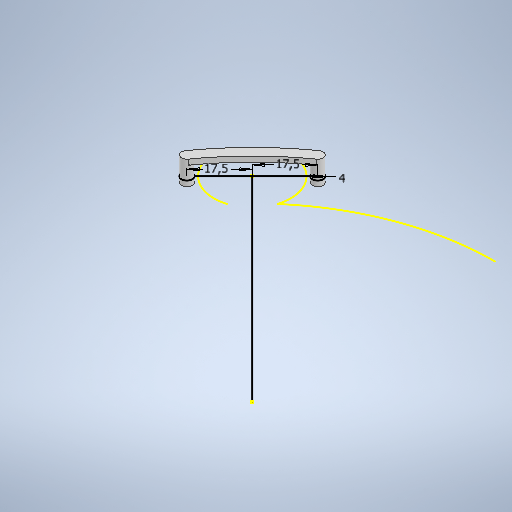
# Autodesk Inventor part: uchwyt
Saved by Autodesk Inventor 2025 (Build 290162000, 162)
## iProperties
Created: 2025-01-24
Part Number: uchwyt
Material: Generic
Document SubType Name: Modeling
Designer: piotr
Density: 1 g/cm^3
Appearance: Default
Author: piotr
Autodesk Inventor part; units mm, degrees
ref_plane "YZ Plane" through (0, 0, 0) normal (1, 0, 0) x (0, 1, 0)
ref_plane "XZ Plane" through (0, 0, 0) normal (0, 1, 0) x (-1, 0, 0)
ref_plane "XY Plane" through (0, 0, 0) normal (0, 0, 1) x (1, 0, 0)
sketch "Sketch3" plane through (0, 0, 0) normal (0, 1, 0) x (-1, 0, 0)
  circle A0 centre (0, 0) radius 91.797
  circle A1 centre (0, 0) radius 110.99
  line L0 (0, 0) -> (110.99, 0)
  line L1 (0, 0) -> (0, -110.99)
  line L2 (91.797, 0) -> (110.99, 0)
  line L3 (0, -45.742) -> (0, -110.99)
  circle A2 centre (0, -101.3935) radius 9.5965
  circle A3 centre (101.3935, 0) radius 9.5965
  circle A4 centre (101.3935, 0) radius 3.125
  circle A5 centre (0, -101.3935) radius 3.125
  circle A6 centre (0, 0) radius 130.99
  line L4 (0, 0) -> (119.0731, -119.0731)
  line L5 (64.9103, -64.9103) -> (73.8174, -73.8174)
  circle A7 centre (73.8174, -73.8174) radius 14.5
  line L6 (76.1136, -88.1344) -> (88.1344, -76.1136)
  line L7 (76.1136, -88.1344) -> (80.7098, -92.7306)
  line L8 (88.1344, -76.1136) -> (92.7306, -80.7098)
  line L9 (80.7098, -92.7306) -> (92.7306, -80.7098)
  line L10 (73.8174, -73.8174) -> (80.7098, -66.9249)
  line L11 (57.15, -95.1455) -> (82.124, -102.0492)
  line L12 (95.1455, -57.15) -> (102.0492, -82.124)
  point P0 (0, -91.797)
  point P1 (103.6367, -80.1113)
  point P2 (69.4945, -59.9767)
  point P3 (87.3148, -68.5194)
  point P4 (68.5194, -87.3148)
  point P5 (59.9767, -69.4945)
  dimension "d9" = 183.594
  dimension "d10" = 221.98
  dimension "d11" = 6.25
  dimension "d14" = 6.25
  dimension "d20" = 20
  dimension "d29" = 45
  dimension "d30" = 12.5965
  dimension "d31" = 29
  dimension "d32" = 17
  dimension "d33" = 6.5
  dimension "d34" = 6.5
  constraints: 26 end point, 9 point on circle, 8 centre point, 5 coincident, 5 perpendicular, 5 point on line, 4 tangent, 2 collinear, 2 symmetric about line, 1 horizontal, 1 midpoint
  measures "d9" diameter of A0
  measures "d10" diameter of A1
  measures "d11" diameter of A4
  measures "d14" diameter of A5
  measures "d20" radial gap between concentric circles of A1 A6
  measures "d29" angle of L4 L1
  measures "d30" distance of L5.start L5.end
  measures "d31" diameter of A7
  measures "d32" distance of L6.start L6.end
  measures "d33" distance of L6.start L7.end
  measures "d34" distance of L6.end L8.end
extrude "Extrusion2" add sketch "Sketch3" along normal blind 3 contours A3 A1 A7 A0 | A3 L0 A4 | L0 A4 A3 | A2 L1 A5 | A0 A7 A1 A2 | L1 A5 A2
extrude "Extrusion3" add sketch "Sketch3" along normal blind 2 contours A1 L12 A6 L4 L9 L8 A7 | A7 L7 L9 L4 A6 L11 A1
fillet "Fillet8" radius 0.99 7 edges at (-62.9566, 2, -91.4071) (-57.15, 1, -95.1455) (-91.4071, 2, -62.9566) (-95.1455, 1, -57.15) (-69.637, 2, -98.5973) (-92.6239, 2, -92.6239) (-98.5973, 2, -69.637)
chamfer "Chamfer2" distance 2 angle 45 1 edges at (-86.7202, 2, -86.7202)
sketch "Sketch5" plane through (0, 3, 0) normal (0, 1, 0) x (1, 0, 0)
  arc A0 (-59.9767, 69.4945) -> (-68.5194, 87.3148) centre (-73.8174, 73.8174) ccw projected
  arc A1 (-87.3148, 68.5194) -> (-69.4945, 59.9767) centre (-73.8174, 73.8174) ccw projected
  arc A2 (0, 91.797) -> (-59.9767, 69.4945) centre (0, 0) ccw projected
  line L0 (0, 0) -> (-73.8174, 73.8174)
  line L1 (-61.443, 86.1917) -> (-73.8174, 73.8174)
  line L2 (-73.8174, 73.8174) -> (-86.1917, 61.443)
  circle A3 centre (-61.443, 86.1917) radius 2
  circle A4 centre (-86.1917, 61.443) radius 2
  dimension "d45" = 17.5
  dimension "d46" = 17.5
  dimension "d47" = 4
  constraints: 6 end point, 2 centre point, 2 coincident, 1 perpendicular, 1 point on line, 1 symmetric about line, 1 other
  measures "d45" distance of L1.start L1.end
  measures "d46" distance of L1.end L2.end
  measures "d47" diameter of A3
extrude "Extrusion4" cut sketch "Sketch5" against normal blind 10
extrude "Extrusion5" add sketch "Sketch5" along normal blind 5 separate body
sketch "Sketch6" plane through (-86.1917, 8, -61.443) normal (0, 1, 0) x (1, 0, 0)
  circle A0 centre (86.1917, -61.443) radius 107.8501
  circle A1 centre (24.7487, 24.7487) radius 2 projected
  circle A2 centre (86.1917, -61.443) radius 103.8501
  circle A3 centre (0, 0) radius 2 projected
  point P0 (1.6286, -1.1609)
  point P1 (25.9097, 23.1202)
  point P2 (23.5878, 26.3773)
  point P3 (-1.6286, 1.1609)
  constraints: 3 tangent, 2 centre point, 2 coincident
extrude "Extrusion6" add sketch "Sketch6" along normal blind 2 contours A1 A2 A3 A0 | A1 | A3 picked at (9.6339, 12.4058) bodies 2
extrude "Extrusion7" add sketch "Sketch5" against normal blind 2 bodies 2
body "Solid2"
body "Solid3"
